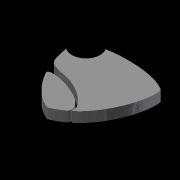
# Autodesk Inventor part: rl shield
Saved by Autodesk Inventor 2018 (Build 220112000, 112)
## iProperties
Created: 2018-05-14
Part Number: rl shield
Material: Aço Inox AISI 304
Document SubType Name: Modeling
Designer: Fábio Ferreira
Density: 7.75 g/cm^3
Sheet Metal Rule: Default_mm
Appearance: Inox
RuleStatus: InUse
BeforeDocSave0: Check Material
BeforeDocSave1: Export_Thickness
Author: Fábio Ferreira
Autodesk Inventor part; units mm, degrees
ref_plane "YZ Plane" through (0, 0, 0) normal (1, 0, 0) x (0, 1, 0)
ref_plane "XZ Plane" through (0, 0, 0) normal (0, 1, 0) x (-1, 0, 0)
ref_plane "XY Plane" through (0, 0, 0) normal (0, 0, 1) x (1, 0, 0)
sketch "Sketch4" plane through (0, 0, 0) normal (0, 0, 1) x (1, 0, 0)
  line L0 (-250, 240.282) -> (250, 240.282) construction
  line L1 (250, 240.282) -> (250, -240.282) construction
  line L2 (250, -240.282) -> (-250, -240.282) construction
  line L3 (-250, -240.282) -> (-250, 240.282) construction
  spline S0 degree 3 poles (-100.5733, 180.0599) (-18.1289, 197.1808) (141.0786, 192.7953) (209.4768, 140.8078) knots 0 0 0 0 1 1 1 1
  spline S1 degree 4 poles (209.4768, 140.8078) (219.2263, 39.4653) (173.7989, -20.0814) (154.7368, -145.8166) (4.6783, -209.1245) knots 0 0 0 0 0 1 1 1 1 1
  spline S2 degree 4 poles (4.6783, -209.1245) (-41.1721, -196.4363) (-172.3084, -114.1593) (-193.9063, 57.1827) (-199.1211, 86.2447) knots 0 0 0 0 0 1 1 1 1 1
  spline S3 degree 4 poles (78.9313, -164.4121) (80.2023, -154.1905) (76.4256, -136.1816) (62.7322, -113.752) (15.649, -74.5367) (-26.5125, -51.7656) (-62.263, -34.3382) (-135.5298, -23.0078) (-168.1733, -11.456) (-175.1008, 1.921) (-181.9892, 13.9507) knots 0 0 0 0 0 0.20248 0.307527 0.423821 0.551794 0.674654 0.784252 1 1 1 1 1
  spline S4 degree 4 poles (-148.0198, -64.2917) (-149.9005, -60.9555) (-146.7781, -54.9625) (-139.1968, -52.3687) (-129.978, -50.8668) (-102.3091, -51.856) (-75.4307, -59.2379) (-59.0818, -61.5978) (19.5287, -91.4105) (59.864, -125.7195) (73.9035, -147.9596) (75.0532, -163.1641) (66.7818, -173.9203) knots 0 0 0 0 0 0.110859 0.16782 0.238431 0.32034 0.433145 0.556354 0.677036 0.793185 1 1 1 1 1
  arc A0 (-199.1211, 86.2447) -> (-100.5733, 180.0599) centre (-158.3351, 142.0684) ccw
  point P0 (0, 0)
  point P1 (0, 240.282)
  point P2 (250, 0)
  point P3 (-2.8391, 189.0369)
  point P4 (123.9149, 176.3847)
  point P5 (204.8802, 59.3886)
  point P6 (181.494, -16.6319)
  point P7 (132.6485, -106.5476)
  point P8 (-49.3817, -180.0894)
  point P9 (-141.2266, -76.0722)
  point P10 (-191.022, 45.65)
  point P11 (78.2312, -149.9094)
  point P12 (72.0281, -132.7953)
  point P13 (55.9746, -110.9345)
  point P14 (18.6852, -79.083)
  point P15 (-24.7132, -53.2255)
  point P16 (-67.4843, -35.9569)
  point P17 (-127.3284, -22.6196)
  point P18 (-159.68, -11.2852)
  point P19 (-172.8121, -0.4015)
  point P20 (-148.0233, -59.0474)
  point P21 (-144.1963, -54.8947)
  point P22 (-139.0258, -52.6962)
  point P23 (-132.3896, -51.5562)
  point P24 (-109.3867, -52.2483)
  point P25 (-81.9055, -57.256)
  point P26 (-59.7984, -62.9559)
  point P27 (17.9712, -95.3711)
  point P28 (56.4602, -126.0196)
  point P29 (69.2027, -144.6024)
  point P30 (72.5925, -158.7334)
  dimension "d23" = 500
  dimension "d27" = 480.564
  constraints: 2 midpoint, 2 point on circle, 1 centre point, 1 horizontal alignment, 1 vertical alignment, 48 other
  measures "d23" distance of L0.start L0.end
  measures "d27" distance of L0.end L1.end
extrude "Extrusion3" add sketch "Sketch4" along normal blind 50 contours S0 S1 S3 S2 A0 | S1 S2 S4
equation "\"BendRadius\" = Thickness"
equation "\"BendReliefWidth\" = Thickness"
equation "\"BendReliefDepth\" = 0.5 * Thickness"
equation "\"CornerReliefSize\" = 4 * Thickness"
equation "\"MinimumRemnant\" = 2 * Thickness"
equation "\"TransitionRadius\" = BendRadius"
equation "\"JacobiRadiusSize\" = BendRadius"
equation "\"GapSize\" = Thickness"
equation "\"Thickness\" = 1.5"
body "Solid4"
